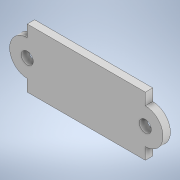
# Autodesk Inventor part: thriftybearingmount_standoff
Saved by Autodesk Inventor 2020 (Build 240168000, 168)
## iProperties
Created: 2020-03-11
Part Number: thriftybearingmount_standoff
Material: Generic
Document SubType Name: Modeling
Designer: srini
Density: 1 g/cm^3
Appearance: Default
Author: srini
Autodesk Inventor part; units mm, degrees
ref_plane "YZ Plane" through (0, 0, 0) normal (1, 0, 0) x (0, 1, 0)
ref_plane "XZ Plane" through (0, 0, 0) normal (0, 1, 0) x (-1, 0, 0)
ref_plane "XY Plane" through (0, 0, 0) normal (0, 0, 1) x (1, 0, 0)
sketch "Sketch1" plane through (0, 0, 0) normal (0, 0, 1) x (1, 0, 0)
  line L0 (-25.4, -12.7) -> (25.4, -12.7)
  line L1 (25.4, -12.7) -> (25.4, 12.7)
  line L2 (25.4, 12.7) -> (-25.4, 12.7)
  line L3 (-25.4, 12.7) -> (-25.4, -12.7)
  line L4 (-25.4, -12.7) -> (25.4, 12.7) construction
  line L5 (25.4, -12.7) -> (-25.4, 12.7) construction
  circle A0 centre (-25.4, 0) radius 7.62
  circle A1 centre (25.4, 0) radius 7.62
  point P0 (0, 0)
  point P1 (-25.4, 7.62)
  point P2 (-25.4, -7.62)
  point P3 (25.4, -7.62)
  point P4 (25.4, 7.62)
  dimension "d0" = 50.8
  dimension "d1" = 25.4
  dimension "d2" = 15.24
  constraints: 12 end point, 4 midpoint, 2 centre point, 2 parallel, 1 equal radius, 1 horizontal, 1 perpendicular
  measures "d0" distance of L1.end L2.end
  measures "d1" distance of L2.end L0.start
  measures "d2" diameter of A0
extrude "Extrusion1" add sketch "Sketch1" along normal blind 3.175
sketch "Sketch2" plane through (0, 0, 3.175) normal (0, 0, 1) x (1, 0, 0)
  arc A0 (-25.4, 7.62) -> (-25.4, -7.62) centre (-25.4, 0) ccw projected
  circle A1 centre (-25.4, 0) radius 2.5781
  arc A2 (25.4, -7.62) -> (25.4, 7.62) centre (25.4, 0) ccw projected
  circle A3 centre (25.4, 0) radius 2.5781
  point P0 (0, 0)
  dimension "d5" = 5.1562
  constraints: 2 centre point, 2 coincident, 1 equal radius
  measures "d5" diameter of A1
extrude "Extrusion2" cut sketch "Sketch2" against normal through all
body "Solid1"
